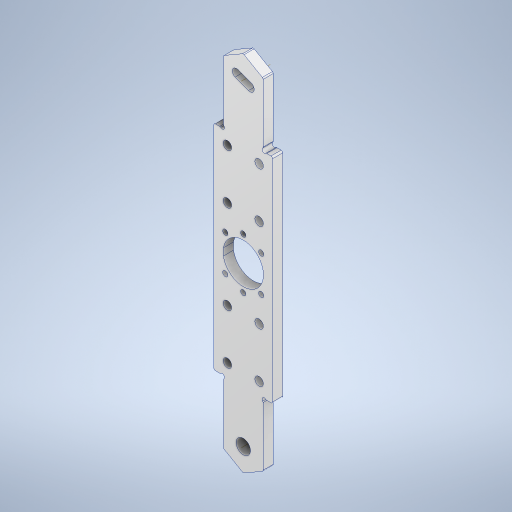
# Autodesk Inventor part: Z-Axis Nut and Bed Plate RevII
Saved by Autodesk Inventor 2024 (Build 280153000, 153)
## iProperties
Created: 2024-08-02
Part Number: Z-Axis Nut and Bed Plate RevII
Material: Aluminum 6061
Document SubType Name: Modeling
Designer: Ishaan
Density: 2.7 g/cm^3
Appearance: Aluminum - Flat
Author: Ishaan
Autodesk Inventor part; units mm, degrees
ref_plane "YZ Plane" through (0, 0, 0) normal (1, 0, 0) x (0, 1, 0)
ref_plane "XZ Plane" through (0, 0, 0) normal (0, 1, 0) x (-1, 0, 0)
ref_plane "XY Plane" through (0, 0, 0) normal (0, 0, 1) x (1, 0, 0)
sketch "Sketch1" plane through (0, 0, 0) normal (0, 0, 1) x (1, 0, 0)
  line L0 (12.5, -107.2169) -> (-12.5, -107.2169)
  line L1 (-12.5, -107.2169) -> (-12.5, 107.2169)
  line L2 (-12.5, 107.2169) -> (12.5, 107.2169)
  line L3 (12.5, 107.2169) -> (12.5, -107.2169)
  line L4 (12.5, -107.2169) -> (-12.5, 107.2169) construction
  line L5 (-12.5, -107.2169) -> (12.5, 107.2169) construction
  line L6 (0, 100) -> (0, -100) construction
  line L7 (-12.5, 107.2169) -> (0, 114.4338)
  line L8 (0, 114.4338) -> (12.5, 107.2169)
  line L9 (12.5, 107.2169) -> (12.5, 92.7831)
  line L10 (12.5, 92.7831) -> (0, 85.5662)
  line L11 (0, 85.5662) -> (-12.5, 92.7831)
  line L12 (-12.5, 92.7831) -> (-12.5, 107.2169)
  line L13 (-12.5, -107.2169) -> (-12.5, -92.7831)
  line L14 (-12.5, -92.7831) -> (0, -85.5662)
  line L15 (0, -85.5662) -> (12.5, -92.7831)
  line L16 (12.5, -92.7831) -> (12.5, -107.2169)
  line L17 (12.5, -107.2169) -> (0, -114.4338)
  line L18 (0, -114.4338) -> (-12.5, -107.2169)
  line L19 (-4.2161, 101.5732) -> (4.2161, 98.4268) construction
  line L20 (-5.1425, 99.0904) -> (3.2896, 95.9441)
  line L21 (5.1425, 100.9096) -> (-3.2896, 104.0559)
  arc A0 (-3.2896, 104.0559) -> (-5.1425, 99.0904) centre (-4.2161, 101.5732) ccw
  arc A1 (3.2896, 95.9441) -> (5.1425, 100.9096) centre (4.2161, 98.4268) ccw
  circle A2 centre (0, -100) radius 4.5
  line L22 (18.5, -67.375) -> (-18.5, -67.375)
  line L23 (-18.5, -67.375) -> (-18.5, 67.375)
  line L24 (-18.5, 67.375) -> (18.5, 67.375)
  line L25 (18.5, 67.375) -> (18.5, -67.375)
  line L26 (18.5, -67.375) -> (-18.5, 67.375) construction
  line L27 (-18.5, -67.375) -> (18.5, 67.375) construction
  circle A3 centre (0, 0) radius 12.7
  point P0 (268, 0)
  point P1 (-12.5, -67.375)
  point P2 (-12.5, 67.375)
  point P3 (12.5, 67.375)
  point P4 (12.5, -67.375)
  point P5 (12.5, -2.245)
  point P6 (-12.5, -2.245)
  point P7 (-12.5, 2.245)
  point P8 (12.5, 2.245)
  dimension "d0" = 25
  dimension "d1" = 268
  dimension "d2" = 200
  dimension "d3" = 5.3
  dimension "d4" = 9
  dimension "d5" = 9
  dimension "d12" = 134.75
  dimension "d13" = 37
  dimension "d43" = 25.4
  constraints: 58 end point, 6 midpoint, 5 parallel, 4 centre point, 4 coincident, 4 point on circle, 4 tangent, 2 collinear, 2 horizontal, 2 perpendicular, 2 point on line, 1 horizontal alignment, 1 vertical, 26 other
  measures "d0" distance of L2.end L1.end
  measures "d1" distance of point (268, 0) point (0, 0)
  measures "d2" distance of L6.start L6.end
  measures "d3" diameter of A1
  measures "d4" distance of L19.start L19.end
  measures "d5" diameter of A2
  measures "d12" distance of L24.end L22.start
  measures "d13" distance between parallel lines of L25 L23
  measures "d43" diameter of A3
extrude "Extrusion1" add sketch "Sketch1" along normal blind 6.35 contours L17 L18 L0 | L0 L1 L14 L15 L3 | L15 L14 L1 L22 L3 | L22 L1 A3 L3 | L3 A3 L24 L25 L22 | L22 L23 L24 L1 A3 | L3 A3 | A3 L1 | A3 L1 L24 L3 | L24 L1 L11 L10 L3 | L10 L11 L1 L2 L3 | L2 L7 L8
sketch "Sketch2" plane through (0, 0, 6.35) normal (0, 0, 1) x (1, 0, 0)
  line L0 (-18.5, 67.375) -> (-18.5, -67.375) projected
  line L1 (-18.5, -67.375) -> (-12.5, -67.375) projected
  line L2 (-12.5, -67.375) -> (-12.5, -107.2169) projected
  line L3 (-12.5, -107.2169) -> (0, -114.4338) projected
  line L4 (0, -114.4338) -> (12.5, -107.2169) projected
  line L5 (12.5, -107.2169) -> (12.5, -67.375) projected
  line L6 (12.5, -67.375) -> (18.5, -67.375) projected
  line L7 (18.5, -67.375) -> (18.5, 67.375) projected
  line L8 (18.5, 67.375) -> (12.5, 67.375) projected
  line L9 (12.5, 67.375) -> (12.5, 107.2169) projected
  line L10 (12.5, 107.2169) -> (0, 114.4338) projected
  line L11 (0, 114.4338) -> (-12.5, 107.2169) projected
  line L12 (-12.5, 107.2169) -> (-12.5, 67.375) projected
  line L13 (-12.5, 67.375) -> (-18.5, 67.375) projected
  arc A0 (-3.2896, 104.0559) -> (-5.1425, 99.0904) centre (-4.2161, 101.5732) ccw projected
  line L14 (-3.2896, 104.0559) -> (5.1425, 100.9096) projected
  arc A1 (3.2896, 95.9441) -> (5.1425, 100.9096) centre (4.2161, 98.4268) ccw projected
  line L15 (3.2896, 95.9441) -> (-5.1425, 99.0904) projected
  circle A2 centre (0, -100) radius 4.5 projected
  circle A3 centre (-13.25, 68.125) radius 1.375
  point P0 (0, 0)
  point P1 (-12.5, 69.2774)
  point P2 (-14.4024, 67.375)
  dimension "d16" = 0.75
  dimension "d17" = 2.75
  dimension "d18" = 0.75
  constraints: 1 centre point
  measures "d16" distance from line of L12 A3.centre
  measures "d17" diameter of A3
  measures "d18" distance from line of A3.centre L13
extrude "Extrusion2" cut sketch "Sketch2" against normal through all contours L13 L12 A3 picked at (-12.4132, 68.57)
mirror "Mirror1" about plane through (0, 0, 0) normal (1, 0, 0) of "Extrusion2"
mirror "Mirror2" about plane through (0, 0, 0) normal (0, 1, 0) of "Extrusion2", "Mirror1"
sketch "Sketch3" plane through (0, 0, 6.35) normal (0, 0, 1) x (1, 0, 0)
  circle A0 centre (0, -100) radius 4.5 projected
  arc A1 (-3.2896, 104.0559) -> (-5.1425, 99.0904) centre (-4.2161, 101.5732) ccw projected
  line L0 (-3.2896, 104.0559) -> (5.1425, 100.9096) projected
  arc A2 (3.2896, 95.9441) -> (5.1425, 100.9096) centre (4.2161, 98.4268) ccw projected
  line L1 (3.2896, 95.9441) -> (-5.1425, 99.0904) projected
  arc A3 (14.4024, -67.375) -> (12.5, -69.2774) centre (13.25, -68.125) ccw projected
  line L2 (14.4024, -67.375) -> (18.5, -67.375) projected
  line L3 (18.5, -67.375) -> (18.5, 67.375) projected
  line L4 (18.5, 67.375) -> (14.4024, 67.375) projected
  arc A4 (12.5, 69.2774) -> (14.4024, 67.375) centre (13.25, 68.125) ccw projected
  line L5 (12.5, 69.2774) -> (12.5, 107.2169) projected
  line L6 (12.5, 107.2169) -> (0, 114.4338) projected
  line L7 (0, 114.4338) -> (-12.5, 107.2169) projected
  line L8 (-12.5, 107.2169) -> (-12.5, 69.2774) projected
  arc A5 (-14.4024, 67.375) -> (-12.5, 69.2774) centre (-13.25, 68.125) ccw projected
  line L9 (-14.4024, 67.375) -> (-18.5, 67.375) projected
  line L10 (-18.5, 67.375) -> (-18.5, -67.375) projected
  line L11 (-18.5, -67.375) -> (-14.4024, -67.375) projected
  arc A6 (-12.5, -69.2774) -> (-14.4024, -67.375) centre (-13.25, -68.125) ccw projected
  line L12 (-12.5, -69.2774) -> (-12.5, -107.2169) projected
  line L13 (-12.5, -107.2169) -> (0, -114.4338) projected
  line L14 (0, -114.4338) -> (12.5, -107.2169) projected
  line L15 (12.5, -107.2169) -> (12.5, -69.2774) projected
  circle A7 centre (0, 0) radius 16 construction
  line L16 (0, 0) -> (11.3137, 11.3137) construction
  line L17 (0, 0) -> (0, 16) construction
  line L18 (0, 0) -> (0, -16) construction
  line L19 (-11.3137, -11.3137) -> (11.3137, -11.3137) construction
  line L20 (11.3137, -11.3137) -> (11.3137, 11.3137) construction
  line L21 (11.3137, 11.3137) -> (-11.3137, 11.3137) construction
  line L22 (-11.3137, 11.3137) -> (-11.3137, -11.3137) construction
  line L23 (-11.3137, -11.3137) -> (11.3137, 11.3137) construction
  line L24 (11.3137, -11.3137) -> (-11.3137, 11.3137) construction
  dimension "d21" = 32
  dimension "d22" = 45
  constraints: 18 end point, 7 coincident, 3 point on circle, 2 midpoint, 2 parallel, 1 centre point, 1 horizontal, 1 perpendicular, 1 point on line, 1 vertical
  measures "d21" diameter of A7
  measures "d22" angle of L16 L17
hole "Hole1" at (-11.3137, 11.3137, 6.35) at (0, 16, 6.35) at (11.3137, 11.3137, 6.35) at (11.3137, -11.3137, 6.35) at (0, -16, 6.35) at (-11.3137, -11.3137, 6.35) direction (0, 0, -1) diameter 3.242 end through all thread size "M4x0.7" class "6H" standard "ANSI Metric M Profile"
sketch "Sketch4" plane through (0, 0, 6.35) normal (0, 0, 1) x (1, 0, 0)
  line L0 (10, -59.375) -> (-10, -59.375) construction
  line L1 (-10, -59.375) -> (-10, 59.375) construction
  line L2 (-10, 59.375) -> (10, 59.375) construction
  line L3 (10, 59.375) -> (10, -59.375) construction
  line L4 (10, -59.375) -> (-10, 59.375) construction
  line L5 (-10, -59.375) -> (10, 59.375) construction
  line L6 (-18.5, -67.375) -> (-14.4024, -67.375) construction
  line L7 (10, -28) -> (-10, -28) construction
  line L8 (-10, -28) -> (-10, 28) construction
  line L9 (-10, 28) -> (10, 28) construction
  line L10 (10, 28) -> (10, -28) construction
  line L11 (10, -28) -> (-10, 28) construction
  line L12 (-10, -28) -> (10, 28) construction
  point P0 (0, 0)
  dimension "d30" = 20
  dimension "d32" = 8
  dimension "d44" = 56
  constraints: 24 end point, 8 coincident, 4 midpoint, 4 parallel, 2 horizontal, 2 perpendicular, 1 point on line
  measures "d30" distance of L1.end L2.end
  measures "d32" distance between parallel lines of L0 L6
  measures "d44" distance between parallel lines of L9 L7
hole "Hole2" at (-10, 59.375, 6.35) at (10, 59.375, 6.35) at (-10, -59.375, 6.35) at (10, -59.375, 6.35) at (-10, 28, 6.35) at (10, 28, 6.35) at (10, -28, 6.35) at (-10, -28, 6.35) direction (0, 0, -1) diameter 5.3 end through all
fillet "Fillet3" radius 1 18 edges at (-18.5, 67.375, 3.175) (-18.5, -67.375, 3.175) (14.4024, -67.375, 3.175) (-14.4024, -67.375, 3.175) (-12.5, -69.2774, 3.175) (18.5, -67.375, 3.175) (12.5, -69.2774, 3.175) (0, -114.4338, 3.175) (12.5, -107.2169, 3.175) (-12.5, -107.2169, 3.175) (18.5, 67.375, 3.175) (-14.4024, 67.375, 3.175) (14.4024, 67.375, 3.175) (0, 114.4338, 3.175) (-12.5, 107.2169, 3.175) (-12.5, 69.2774, 3.175) (12.5, 69.2774, 3.175) (12.5, 107.2169, 3.175)
equation "\"d18\" = d16"
body "Solid1"
